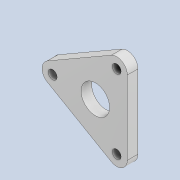
# Autodesk Inventor part: 最終段小ギア軸受け
Saved by Autodesk Inventor 2020.4 (Build 244396000, 396)
## iProperties
Created: 2021-04-23
Part Number: 最終段小ギア軸受け
Material: アルミニウム 2014-T4
Document SubType Name: Modeling
Designer: happy
Density: 2.8 g/cm^3
Appearance: サテン
Author: happy
Autodesk Inventor part; units mm, degrees
ref_plane "YZ Plane" through (0, 0, 0) normal (1, 0, 0) x (0, 1, 0)
ref_plane "XZ Plane" through (0, 0, 0) normal (0, 1, 0) x (-1, 0, 0)
ref_plane "XY Plane" through (0, 0, 0) normal (0, 0, 1) x (1, 0, 0)
sketch "スケッチ1" plane through (0, 0, 0) normal (0, 0, 1) x (1, 0, 0)
  circle A0 centre (116.7187, 16.8502) radius 1.5 construction
  circle A1 centre (116.7187, 16.8502) radius 3
  circle A2 centre (134.7937, 6.4146) radius 3
  circle A3 centre (134.7937, 27.2858) radius 3
  line L0 (115.2187, 19.4483) -> (133.2937, 29.8839)
  line L1 (137.7937, 27.2858) -> (137.7937, 6.4146)
  line L2 (133.2937, 3.8165) -> (115.2187, 14.2522)
  circle A4 centre (116.7187, 16.8502) radius 1.25
  circle A5 centre (134.7937, 6.4146) radius 1.25
  circle A6 centre (134.7937, 27.2858) radius 1.25
  circle A7 centre (128.7687, 16.8502) radius 4.025
  point P0 (0, 0)
  point P1 (0, 0)
  dimension "d4" = 6
  dimension "d5" = 360
  dimension "d6" = 2.5
  dimension "d7" = 360
  constraints: 8 centre point, 6 end point, 6 point on circle, 6 tangent, 2 coincident, 18 other
  measures "d4" diameter of A1
  measures "d6" diameter of A4
extrude "押し出し1" add sketch "スケッチ1" along normal blind 3
